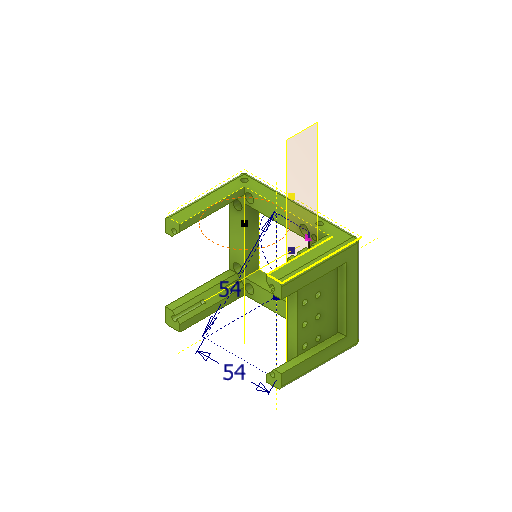
# Autodesk Inventor part: 20_Cube_Insert_Beamsplittercube_motorized_cube_base
Saved by Autodesk Inventor 2022 (Build 260153000, 153)
## iProperties
Created: 2019-07-01
Part Number: 20_Cube_Insert_Beamsplittercube_motorized_cube_base
Material: Generic
Document SubType Name: Modeling
Designer: diederichbenedict
Density: 1 g/cm^3
Appearance: IPHT_Grün
Author: diederichbenedict
Autodesk Inventor part; units mm, degrees
ref_plane "YZ Plane" through (0, 0, 0) normal (1, 0, 0) x (0, 1, 0)
ref_plane "XZ Plane" through (0, 0, 0) normal (0, 1, 0) x (-1, 0, 0)
sketch "Sketch1" plane through (0, 0, 0) normal (0, 0, 1) x (1, 0, 0)
  line L0 (-24.9, 24.9) -> (24.9, 24.9)
  line L1 (24.9, 24.9) -> (24.9, -24.9)
  line L2 (24.9, -24.9) -> (-24.9, -24.9)
  line L3 (-24.9, -24.9) -> (-24.9, 24.9)
  line L4 (-24.9, 24.9) -> (24.9, -24.9) construction
  line L5 (24.9, 24.9) -> (-24.9, -24.9) construction
  line L6 (17.05, 17.05) -> (-17.05, 17.05)
  line L7 (-17.05, 17.05) -> (-17.05, -17.05)
  line L8 (-17.05, -17.05) -> (17.05, -17.05)
  line L9 (17.05, -17.05) -> (17.05, 17.05)
  line L10 (24.9, 24.9) -> (36.9, 24.9)
  line L11 (36.9, 24.9) -> (36.9, -24.9)
  line L12 (36.9, -24.9) -> (24.9, -24.9)
  line L13 (24.9, -24.9) -> (24.9, 24.9)
  point P0 (0, 0)
  dimension "d0" = 49.8
  dimension "d1" = 49.8
  dimension "d2" = 7.85
  dimension "d124" = 12
  constraints: 28 end point, 6 parallel, 3 perpendicular, 2 horizontal, 2 midpoint, 3 other
  measures "d0" distance of L1.end L2.end
  measures "d1" distance of L0.end L1.end
  measures "d2" distance between parallel lines of L0 L6
  measures "d124" distance of L11.end L12.end
extrude "Extrusion1" add sketch "Sketch1" along normal blind 7.7
sketch "Sketch2" plane through (0, 0, 7.7) normal (0, 0, 1) x (1, 0, 0)
  line L0 (17.05, 17.05) -> (17.05, -17.05) projected
  line L1 (17.05, -17.05) -> (-17.05, -17.05) projected
  line L2 (-17.05, -17.05) -> (-17.05, 17.05) projected
  line L3 (-17.05, 17.05) -> (17.05, 17.05) projected
  line L4 (36.9, 24.9) -> (-24.9, 24.9) projected
  line L5 (-24.9, 24.9) -> (-24.9, -24.9) projected
  line L6 (-24.9, -24.9) -> (36.9, -24.9) projected
  line L7 (17.05, -17.05) -> (24.9, -17.05)
  line L8 (24.9, -17.05) -> (24.9, -24.9)
  line L9 (24.9, -24.9) -> (17.05, -24.9)
  line L10 (17.05, -24.9) -> (17.05, -17.05)
  line L11 (17.05, 17.05) -> (-17.05, 17.05) projected
  line L12 (24.9, 24.9) -> (17.05, 24.9)
  line L13 (17.05, 24.9) -> (17.05, 17.05)
  line L14 (17.05, 17.05) -> (24.9, 17.05)
  line L15 (24.9, 17.05) -> (24.9, 24.9)
  line L16 (-24.9, -24.9) -> (-17.05, -24.9)
  line L17 (-17.05, -24.9) -> (-17.05, -17.05)
  line L18 (-17.05, -17.05) -> (-24.9, -17.05)
  line L19 (-24.9, -17.05) -> (-24.9, -24.9)
  line L20 (-24.9, 24.9) -> (-17.05, 24.9)
  line L21 (-17.05, 24.9) -> (-17.05, 17.05)
  line L22 (-17.05, 17.05) -> (-24.9, 17.05)
  line L23 (-24.9, 17.05) -> (-24.9, 24.9)
  line L24 (36.9, -24.9) -> (36.9, 24.9) projected
  line L25 (36.9, -24.9) -> (29.05, -24.9)
  line L26 (29.05, -24.9) -> (29.05, -17.05)
  line L27 (29.05, -17.05) -> (36.9, -17.05)
  line L28 (36.9, -17.05) -> (36.9, -24.9)
  line L29 (36.9, 24.9) -> (-24.9, 24.9) projected
  line L30 (36.9, 24.9) -> (29.05, 24.9)
  line L31 (29.05, 24.9) -> (29.05, 17.05)
  line L32 (29.05, 17.05) -> (36.9, 17.05)
  line L33 (36.9, 17.05) -> (36.9, 24.9)
  point P0 (0, 0)
  dimension "d125" = 7.85
  constraints: 48 end point, 12 parallel, 6 horizontal, 6 perpendicular
  measures "d125" distance between parallel lines of L28 L26
extrude "Extrusion2" add sketch "Sketch2" along normal blind 34.4 contours L22 L5 L4 L21 | L17 L6 L5 L18 | L4 L24 L32 L31 | L26 L27 L24 L6
sketch "Sketch3" plane through (0, 0, 0) normal (0, 0, -1) x (-1, 0, 0)
  line L0 (24.9, -24.9) -> (24.9, 24.9) construction
  line L1 (-36.9, 24.9) -> (24.9, 24.9) construction
  line L2 (-36.9, -24.9) -> (24.9, -24.9) construction
  line L3 (-24.9, 24.9) -> (-24.9, -24.9) construction
  point P0 (20, 20)
  point P1 (20, -20)
  point P2 (-20, -20)
  point P3 (-20, 20)
  dimension "d96" = 4.9
  dimension "d97" = 4.9
  dimension "d98" = 4.9
  dimension "d99" = 4.9
  dimension "d100" = 4.9
  dimension "d101" = 4.9
  dimension "d140" = 4.9
  dimension "d141" = 4.9
  measures "d96" distance from line of point (20, 20) L0
  measures "d97" distance from line of point (20, -20) L0
  measures "d98" distance from line of point (20, -20) L2
  measures "d99" distance from line of point (-20, -20) L2
  measures "d100" distance from line of point (-20, -20) L3
  measures "d101" distance from line of point (-20, 20) L3
  measures "d140" distance from line of point (20, 20) L1
  measures "d141" distance from line of L1 point (-20, 20)
hole "Hole1" at (-20, 20, 0) at (-20, -20, 0) at (20, -20, 0) at (20, 20, 0) direction (0, 0, 1) diameter 2.8 depth 16 tip angle 118 counterbore diameter 5.5 counterbore depth 3.1
sketch "Sketch4" plane through (-24.9, 24.9, 0) normal (0, 1, 0) x (1, 0, 0)
  line L0 (61.8, 0) -> (0, 0) construction
  line L1 (0, 0) -> (0, -42.1) construction
  line L2 (7.85, -42.1) -> (0, -42.1) construction
  line L3 (7.85, -7.7) -> (7.85, -42.1) construction
  line L4 (53.95, -7.7) -> (7.85, -7.7) construction
  circle A0 centre (24.9, -24.75) radius 17.05 construction
  line L5 (53.95, -7.7) -> (53.95, -42.1) projected
  line L6 (61.8, -42.1) -> (53.95, -42.1) projected
  line L7 (61.8, 0) -> (61.8, -42.1) projected
  point P0 (24.9, 0)
  constraints: 2 tangent, 1 centre point
sketch "Sketch5" plane through (0, 0, 0) normal (0, 0, -1) x (-1, 0, 0)
  line L0 (-17.05, -17.05) -> (-17.05, 17.05) construction
  line L1 (-17.05, 17.05) -> (17.05, 17.05) construction
  line L2 (17.05, 17.05) -> (17.05, -17.05) construction
  line L3 (17.05, -17.05) -> (-17.05, -17.05) construction
  circle A0 centre (0, 0) radius 17.05 construction
  point P0 (0, 0)
  constraints: 3 tangent, 1 centre point
fillet "Fillet1" radius 2 8 edges at (-24.9, -24.9, 21.05) (-24.9, 24.9, 21.05) (-24.9, 0, 0) (6, -24.9, 0) (6, 24.9, 0) (36.9, -24.9, 21.05) (36.9, 24.9, 21.05) (36.9, 0, 0)
sketch "Sketch6" plane through (0, 0, 42.1) normal (0, 0, 1) x (1, 0, 0)
  arc A0 (-22.9, 24.9) -> (-24.9, 22.9) centre (-22.9, 22.9) ccw projected
  line L0 (-24.9, 22.9) -> (-24.9, 17.05) projected
  line L1 (-24.9, 17.05) -> (-17.05, 17.05) projected
  line L2 (-17.05, 17.05) -> (-17.05, 24.9) projected
  line L3 (-17.05, 24.9) -> (-22.9, 24.9) projected
  arc A1 (24.9, 22.9) -> (22.9, 24.9) centre (22.9, 22.9) ccw projected
  line L4 (22.9, 24.9) -> (17.05, 24.9) projected
  line L5 (17.05, 24.9) -> (17.05, 17.05) projected
  line L6 (17.05, 17.05) -> (24.9, 17.05) projected
  line L7 (24.9, 17.05) -> (24.9, 22.9) projected
  arc A2 (22.9, -24.9) -> (24.9, -22.9) centre (22.9, -22.9) ccw projected
  line L8 (24.9, -22.9) -> (24.9, -17.05) projected
  line L9 (24.9, -17.05) -> (17.05, -17.05) projected
  line L10 (17.05, -17.05) -> (17.05, -24.9) projected
  line L11 (17.05, -24.9) -> (22.9, -24.9) projected
  arc A3 (-24.9, -22.9) -> (-22.9, -24.9) centre (-22.9, -22.9) ccw projected
  line L12 (-22.9, -24.9) -> (-17.05, -24.9) projected
  line L13 (-17.05, -24.9) -> (-17.05, -17.05) projected
  line L14 (-17.05, -17.05) -> (-24.9, -17.05) projected
  line L15 (-24.9, -17.05) -> (-24.9, -22.9) projected
  line L16 (0, 38.1838) -> (54, 38.1838) construction
  line L17 (21.2752, 17.05) -> (17.05, 21.2752)
  line L18 (17.05, 24.9) -> (17.05, 17.05) projected
  line L19 (17.05, 21.2752) -> (17.05, 17.05)
  line L20 (17.05, 17.05) -> (21.2752, 17.05)
  line L21 (-17.05, 24.9) -> (-17.05, 17.05) projected
  line L22 (-17.05, 17.05) -> (-17.05, 21.2752)
  line L23 (-17.05, 21.2752) -> (-21.2752, 17.05)
  line L24 (-17.05, 21.2752) -> (-11.0747, 21.2752) construction
  line L25 (-17.05, -17.05) -> (-17.05, 17.05) projected
  line L26 (-21.2752, 17.05) -> (-17.05, 17.05)
  line L27 (-17.05, 17.05) -> (-21.2752, 17.05)
  line L28 (17.05, -17.05) -> (17.05, -24.9) projected
  line L29 (17.05, -17.05) -> (21.2752, -17.05)
  line L30 (24.9, -17.05) -> (17.05, -17.05) projected
  line L31 (21.2752, -17.05) -> (17.05, -21.2752)
  line L32 (17.05, -17.05) -> (17.05, -21.2752)
  line L33 (-17.05, -17.05) -> (-21.2752, -17.05)
  line L34 (-17.05, -17.05) -> (-17.05, -24.9) projected
  line L35 (-17.05, -17.05) -> (-17.05, -21.2752)
  line L36 (-21.2752, -17.05) -> (-17.05, -21.2752)
  line L37 (22.9, 22.9) -> (24.9, 22.9) construction
  line L38 (-22.9, -22.9) -> (22.9, 22.9) construction
  line L39 (-22.9, -22.9) -> (34.9, -22.9) construction
  line L40 (34.9, 22.9) -> (-22.9, 22.9) construction
  line L41 (22.9, -22.9) -> (-22.9, 22.9) construction
  line L42 (29.05, -17.05) -> (29.05, -24.9) projected
  line L43 (29.05, -24.9) -> (34.9, -24.9) projected
  line L44 (36.9, -22.9) -> (36.9, -17.05) projected
  line L45 (36.9, -17.05) -> (29.05, -17.05) projected
  line L46 (36.9, 17.05) -> (36.9, 22.9) projected
  line L47 (34.9, 24.9) -> (29.05, 24.9) projected
  line L48 (29.05, 24.9) -> (29.05, 17.05) projected
  line L49 (29.05, 17.05) -> (36.9, 17.05) projected
  line L50 (29.05, 24.9) -> (29.05, 17.05) projected
  line L51 (29.05, 21.2752) -> (32.975, 17.05)
  line L52 (36.9, 17.05) -> (29.05, 17.05) projected
  line L53 (29.05, -17.05) -> (29.05, -24.9) projected
  line L54 (29.05, -21.2752) -> (32.975, -17.05)
  line L55 (29.05, -17.05) -> (36.9, -17.05) projected
  arc A4 (34.9, -24.9) -> (36.9, -22.9) centre (34.9, -22.9) ccw projected
  arc A5 (36.9, 22.9) -> (34.9, 24.9) centre (34.9, 22.9) ccw projected
  point P0 (36.9, 22.9)
  dimension "d111" = 0
  dimension "d120" = 54.2
  dimension "d121" = 54.2
  constraints: 38 end point, 11 point on line, 3 collinear, 3 perpendicular, 2 horizontal, 2 midpoint, 1 equal length, 1 parallel, 1 vertical, 1 other
  measures "d111" vertical distance of L35.end L31.end
  measures "d120" distance between parallel lines of L31 L23
  measures "d121" distance between parallel lines of L36 L17
extrude "Extrusion3" cut sketch "Sketch6" against normal up to surface (34.4 mm away) contours L2 L1 L23 | L10 L9 L31 | L14 L13 L36 | L45 L54 L42 | L49 L48 L51
sketch "Sketch8" plane through (17.05, -24.9, 7.7) normal (-1, 0, 0) x (0, 0, 1)
  line L0 (-4.0838, 41.95) -> (0, 41.95) construction
  line L1 (-4.0838, 7.85) -> (0.1503, 7.85) construction
  line L2 (0.1503, 7.85) -> (0.1503, 3.6159) construction
  line L3 (-4.0838, 7.85) -> (0.1503, 3.6159)
  line L4 (0.1503, 3.6159) -> (0.1503, 7.85)
  line L5 (0.1503, 7.85) -> (-4.0838, 7.85)
  line L6 (-4.0838, 41.95) -> (0, 46.0338)
  line L7 (-4.0838, 41.95) -> (1.6916, 41.95) construction
  line L8 (0.1503, 7.85) -> (0, 41.95)
  line L9 (0, 46.0338) -> (0, 41.95)
  line L10 (0, 41.95) -> (-4.0838, 41.95)
  line L11 (-6, 2) -> (-6, 47.8)
  line L12 (55.2338, 24.9) -> (17.05, 63.0838) construction
  line L13 (17.05, 63.0838) -> (-21.1338, 24.9) construction
  line L14 (-21.1338, 24.9) -> (17.05, -13.2838) construction
  line L15 (17.05, -13.2838) -> (55.2338, 24.9) construction
  line L16 (55.2338, 24.9) -> (-21.1338, 24.9) construction
  line L17 (17.05, 63.0838) -> (17.05, -13.2838) construction
  line L18 (-36.4073, 24.9) -> (70.5073, 24.9) construction
  line L19 (17.05, -28.5573) -> (17.05, 78.3573) construction
  line L20 (0, 41.95) -> (0, 46.1752) construction
  line L21 (0, 7.85) -> (-4.0972, 7.85) construction
  line L22 (-4.0972, 41.95) -> (-4.0972, 7.85) construction
  line L23 (0, 41.95) -> (-4.0972, 41.95) construction
  line L24 (0, 7.85) -> (0, 41.95) construction
  point P0 (-2.4341, 8)
  point P1 (0, 5.414)
  point P2 (17.05, 24.9)
  point P3 (17.05, 24.9)
  point P4 (17.05, 24.9)
  point P5 (0, 43.5346)
  dimension "d122" = 54
  dimension "d123" = 54
  constraints: 32 end point, 6 midpoint, 4 collinear, 3 horizontal, 2 parallel, 2 perpendicular, 2 vertical, 1 equal length, 1 point on line, 6 other
  measures "d122" distance of L12.start L12.end
  measures "d123" distance of L14.end L12.start
ref_plane "Work Plane1" through (-20.32, -18.034, 19.8181) normal (-1, 0, 0) x (0, 0, 1)
sketch "Sketch9" plane through (0, 0, 42.1) normal (0, 0, 1) x (1, 0, 0)
  arc A0 (19.6906, 18.6346) -> (18.6346, 19.6906) centre (20, 20) ccw projected
  arc A1 (18.6346, -19.6906) -> (19.6906, -18.6346) centre (20, -20) ccw projected
  arc A2 (-19.6906, -18.6346) -> (-18.6346, -19.6906) centre (-20, -20) ccw projected
  arc A3 (-18.6346, 19.6906) -> (-19.6906, 18.6346) centre (-20, 20) ccw projected
  line L0 (29.05, 21.2752) -> (32.975, 17.05) projected
  line L1 (32.975, 17.05) -> (36.9, 17.05) projected
  line L2 (36.9, 17.05) -> (36.9, 22.9) projected
  arc A4 (36.9, 22.9) -> (34.9, 24.9) centre (34.9, 22.9) ccw projected
  line L3 (34.9, 24.9) -> (29.05, 24.9) projected
  line L4 (29.05, 24.9) -> (29.05, 21.2752) projected
  line L5 (32.975, -17.05) -> (29.05, -21.2752) projected
  line L6 (29.05, -21.2752) -> (29.05, -24.9) projected
  line L7 (29.05, -24.9) -> (34.9, -24.9) projected
  arc A5 (34.9, -24.9) -> (36.9, -22.9) centre (34.9, -22.9) ccw projected
  line L8 (36.9, -22.9) -> (36.9, -17.05) projected
  line L9 (36.9, -17.05) -> (32.975, -17.05) projected
  circle A6 centre (31.975, -19.6906) radius 1.4
  circle A7 centre (31.975, 20.0567) radius 1.4
  dimension "d126" = 2.8
  dimension "d127" = 2.8
  constraints: 2 centre point
  measures "d126" diameter of A6
  measures "d127" diameter of A7
hole "Hole2" at (20, 20, 42.1) at (-20, 20, 42.1) at (20, -20, 42.1) at (-20, -20, 42.1) at (31.975, -19.6906, 42.1) at (31.975, 20.0567, 42.1) direction (0, 0, -1) diameter 2.8 depth 15 tip angle 118
sketch "Sketch12" plane through (-17.05, -24.9, 7.7) normal (0, -1, 0) x (1, 0, 0)
  line L0 (-7.85, 34.4) -> (-7.85, -5.7) construction
  line L1 (-5.85, -7.7) -> (51.95, -7.7) construction
  line L2 (41.95, 0) -> (41.95, 34.4) construction
  line L3 (-5.85, -7.7) -> (51.95, -7.7) construction
  point P0 (-2.3319, -8)
  point P1 (36.1319, -8)
  point P2 (41.95, -5.7)
  point P3 (-2.95, -2.8)
  point P4 (37.05, -2.8)
  point P5 (37.6681, -8)
  point P6 (39.95, -7.7)
  point P7 (53.95, -7.7)
  dimension "d91" = 4.9
  dimension "d92" = 4.9
  dimension "d93" = 4.9
  dimension "d94" = 4.9
  constraints: 2 other
  measures "d91" distance from line of point (-2.95, -2.8) L0
  measures "d94" distance from line of L2 point (37.05, -2.8)
hole "Hole5" at (-20, -24.9, 4.9) at (20, -24.9, 4.9) direction (0, 1, 0) diameter 2.9 depth 6.5 tip angle 118
sketch "Sketch13" plane through (-24.9, -17.05, 7.7) normal (-1, 0, 0) x (0, 0, 1)
  circle A0 centre (-2.8, 37.05) radius 1.45 projected
  circle A1 centre (-2.8, -2.95) radius 1.45 projected
  point P0 (-3.6423, -3.1)
  constraints: 1 other
hole "Hole6" at (-24.9, 20, 4.9) at (-24.9, -20, 4.9) direction (1, 0, 0) diameter 2.9 depth 6.5 tip angle 118
sketch "Sketch14" plane through (-17.05, 24.9, 7.7) normal (0, 1, 0) x (1, 0, 0)
  circle A0 centre (37.05, 2.8) radius 1.45 projected
  circle A1 centre (-2.95, 2.8) radius 1.45 projected
hole "Hole7" at (-20, 24.9, 4.9) at (20, 24.9, 4.9) direction (0, -1, 0) diameter 2.9 depth 6.5 tip angle 118
sketch "Sketch15" plane through (0, 0, 0) normal (0, 0, -1) x (-1, 0, 0)
  line L0 (-17.05, -17.05) -> (-17.05, 17.05) construction
  line L1 (-17.05, 17.05) -> (17.05, 17.05) construction
  line L2 (17.05, 17.05) -> (17.05, -17.05) construction
  line L3 (17.05, -17.05) -> (-17.05, -17.05) construction
  circle A0 centre (20, -20) radius 2.75 construction
  circle A1 centre (-20, -20) radius 2.75 construction
  line L4 (-34.9, 22.9) -> (22.9, 22.9) construction
  line L5 (22.9, -22.9) -> (-34.9, -22.9) construction
  line L6 (22.9, 22.9) -> (22.9, -22.9) construction
  line L7 (17.05, 21.1338) -> (-17.05, 21.1338) construction
  line L8 (-34.9, -22.9) -> (-34.9, 22.9) projected
  point P0 (0, 0)
  point P1 (-20.8, -14.5)
  point P2 (-14.5, -20.8)
  point P3 (14.5, -20.8)
  point P4 (20.8, -14.5)
  point P5 (20.8, 14.5)
  point P6 (14.5, 20.8)
  point P7 (-14.5, 20.8)
  point P8 (-20.8, 14.5)
hole "Hole8" at (14.5, -20.8, 0) at (20.8, -14.5, 0) at (-14.5, -20.8, 0) at (-20.8, -14.5, 0) at (-20.8, 14.5, 0) at (-14.5, 20.8, 0) at (14.5, 20.8, 0) at (20.8, 14.5, 0) direction (0, 0, 1) diameter 4.7 end through all
ref_plane "Arbeitsebene4" through (27.26, 5.1412, 21.6068) normal (1, 0, 0) x (0, -1, 0)
sketch "Skizze17" plane through (27.26, 5.1412, 21.6068) normal (1, 0, 0) x (0, -1, 0)
  circle A0 centre (-46.675, -3.55) radius 1.57 projected
  circle A1 centre (-46.675, 3.55) radius 1.57 projected
  line L0 (23.225, -7.55) -> (12.725, -7.55) projected
  line L1 (23.225, 7.55) -> (23.225, -7.55) projected
  line L2 (12.725, 7.55) -> (23.225, 7.55) projected
  line L3 (12.725, 5.55) -> (12.725, 7.55) projected
  line L4 (4.725, 5.55) -> (12.725, 5.55) projected
  line L5 (4.725, 7.55) -> (4.725, 5.55) projected
  line L6 (4.725, 7.55) -> (-51.175, 7.55) projected
  line L7 (-51.175, 7.55) -> (-51.175, 5.55) projected
  line L8 (-51.175, 5.55) -> (-59.175, 5.55) projected
  line L9 (-59.175, 5.55) -> (-59.175, 7.55) projected
  line L10 (-59.175, 7.55) -> (-69.675, 7.55) projected
  line L11 (-69.675, 7.55) -> (-69.675, -7.55) projected
  line L12 (-69.675, -7.55) -> (-59.175, -7.55) projected
  line L13 (-59.175, -7.55) -> (-59.175, -5.55) projected
  line L14 (-59.175, -5.55) -> (-51.175, -5.55) projected
  line L15 (-51.175, -5.55) -> (-51.175, -7.55) projected
  line L16 (4.725, -7.55) -> (-51.175, -7.55) projected
  line L17 (4.725, -5.55) -> (4.725, -7.55) projected
  line L18 (12.725, -5.55) -> (4.725, -5.55) projected
  line L19 (12.725, -7.55) -> (12.725, -5.55) projected
  circle A2 centre (0.225, 3.55) radius 1.57 construction
  circle A3 centre (0.225, -3.55) radius 1.57 construction
  line L20 (30.0412, 13.9068) -> (30.0412, -20.4932) projected
  line L21 (-19.7588, 13.9068) -> (-16.134, 13.9068) projected
  line L22 (30.0412, -7.55) -> (-19.7588, -7.55)
  line L23 (-19.7588, -7.55) -> (-19.7588, 13.9068)
  line L24 (-19.7588, 13.9068) -> (30.0412, 13.9068)
  line L25 (30.0412, 13.9068) -> (30.0412, -7.55)
  circle A4 centre (0.225, -3.55) radius 1.4
  circle A5 centre (0.225, 3.55) radius 1.4
  circle A6 centre (-46.675, -3.55) radius 1.57 projected
  circle A7 centre (-46.675, 3.55) radius 1.57 projected
  line L26 (23.225, -7.55) -> (12.725, -7.55) projected
  line L27 (23.225, 7.55) -> (23.225, -7.55) projected
  line L28 (12.725, 7.55) -> (23.225, 7.55) projected
  line L29 (12.725, 5.55) -> (12.725, 7.55) projected
  line L30 (4.725, 5.55) -> (12.725, 5.55) projected
  line L31 (4.725, 7.55) -> (4.725, 5.55) projected
  line L32 (4.725, 7.55) -> (-51.175, 7.55) projected
  line L33 (-51.175, 7.55) -> (-51.175, 5.55) projected
  line L34 (-51.175, 5.55) -> (-59.175, 5.55) projected
  line L35 (-59.175, 5.55) -> (-59.175, 7.55) projected
  line L36 (-59.175, 7.55) -> (-69.675, 7.55) projected
  line L37 (-69.675, 7.55) -> (-69.675, -7.55) projected
  line L38 (-69.675, -7.55) -> (-59.175, -7.55) projected
  line L39 (-59.175, -7.55) -> (-59.175, -5.55) projected
  line L40 (-59.175, -5.55) -> (-51.175, -5.55) projected
  line L41 (-51.175, -5.55) -> (-51.175, -7.55) projected
  line L42 (4.725, -7.55) -> (-51.175, -7.55) projected
  line L43 (4.725, -5.55) -> (4.725, -7.55) projected
  line L44 (12.725, -5.55) -> (4.725, -5.55) projected
  line L45 (12.725, -7.55) -> (12.725, -5.55) projected
  circle A8 centre (0.225, 3.55) radius 1.57 construction
  circle A9 centre (0.225, -3.55) radius 1.57 construction
  circle A10 centre (-9.775, -3.55) radius 1.4
  circle A11 centre (-9.775, 3.55) radius 1.4
  line L46 (20.0412, -7.55) -> (-29.7588, -7.55)
  circle A12 centre (-19.775, -3.55) radius 1.4
  circle A13 centre (-19.775, 3.55) radius 1.4
  line L47 (10.0412, -7.55) -> (-39.7588, -7.55)
  circle A14 centre (10.225, -3.55) radius 1.4
  circle A15 centre (10.225, 3.55) radius 1.4
  line L48 (40.0412, -7.55) -> (-9.7588, -7.55)
  circle A16 centre (0.225, -3.55) radius 1.4
  circle A17 centre (0.225, 3.55) radius 1.4
  line L49 (30.0412, -7.55) -> (-19.7588, -7.55)
  circle A18 centre (-9.775, -3.55) radius 1.4
  circle A19 centre (-9.775, 3.55) radius 1.4
  line L50 (20.0412, -7.55) -> (-29.7588, -7.55)
  circle A20 centre (20.225, -3.55) radius 1.4
  circle A21 centre (20.225, 3.55) radius 1.4
  line L51 (50.0412, -7.55) -> (0.2412, -7.55)
  circle A22 centre (10.225, -3.55) radius 1.4
  circle A23 centre (10.225, 3.55) radius 1.4
  line L52 (40.0412, -7.55) -> (-9.7588, -7.55)
  circle A24 centre (0.225, -3.55) radius 1.4
  circle A25 centre (0.225, 3.55) radius 1.4
  line L53 (30.0412, -7.55) -> (-19.7588, -7.55)
  circle A26 centre (30.225, -3.55) radius 1.4
  circle A27 centre (30.225, 3.55) radius 1.4
  line L54 (60.0412, -7.55) -> (10.2412, -7.55)
  circle A28 centre (20.225, -3.55) radius 1.4
  circle A29 centre (20.225, 3.55) radius 1.4
  line L55 (50.0412, -7.55) -> (0.2412, -7.55)
  circle A30 centre (10.225, -3.55) radius 1.4
  circle A31 centre (10.225, 3.55) radius 1.4
  line L56 (40.0412, -7.55) -> (-9.7588, -7.55)
  point P0 (5.1412, 21.6068)
  point P1 (30.0412, 2.1621)
  point P2 (30.0412, 4.9379)
  point P3 (-19.7588, 4.9499)
  point P4 (-19.7588, 2.1501)
  point P5 (-19.7588, -2.1501)
  point P6 (-19.7588, -4.9499)
  point P7 (-19.7588, -7.55)
  point P8 (12.725, -7.55)
  point P9 (30.0412, -4.9379)
  point P10 (30.0412, -2.1621)
  dimension "d128" = 2.8
  dimension "d129" = 2.8
  dimension "d132" = 10
  dimension "d135" = 10
  constraints: 30 end point, 24 centre point, 24 coincident, 3 horizontal, 2 collinear, 2 parallel, 1 perpendicular, 1 point on line, 119 other
  measures "d128" diameter of A4
  measures "d129" diameter of A5
  measures "d132" distance of A3.centre point (-9.775, -3.55)
  measures "d135" distance of A3.centre point (10.225, -3.55)
extrude "Extrusion6" add sketch "Skizze17" along normal blind 5 contours L0 L19 L18 L17 L16 L23 A12 A13 L6 L5 L4 L3 L2 L1 | L1 L2 L3 L4 L5 L6 L23 L21 L24 L20 A27 A26 L22 | L22 L17 L18 L19
equation "\"d1\" = d0"
equation "\"d96\" = d_1"
equation "\"d97\" = d_1"
equation "\"d98\" = d_1"
equation "\"d99\" = d_1"
equation "\"d100\" = d_1"
equation "\"d101\" = d_1"
equation "\"d121\" = d120"
equation "\"d_1\" = 4.9"
body "Solid1"
